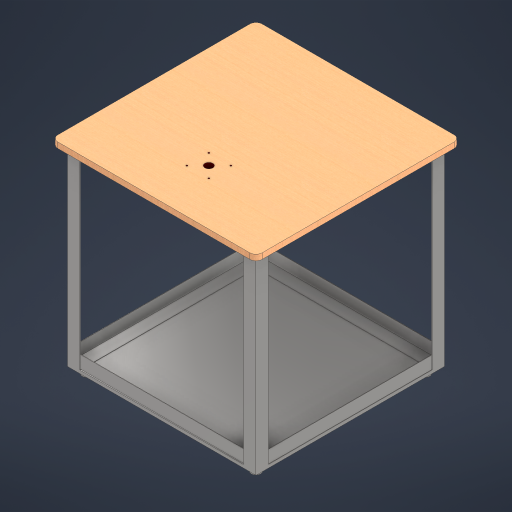
# Autodesk Inventor part: Foundation-Base
Saved by Autodesk Inventor 2023 (Build 270158000, 158)
## iProperties
Created: 2023-09-14
Part Number: Foundation-Base
Material: Steel, Mild
Document SubType Name: Modeling
Designer: Abhinav
Density: 7.85 g/cm^3
Appearance: Semi-Polished
Author: Abhinav
Autodesk Inventor part; units mm, degrees
ref_plane "YZ Plane" through (0, 0, 0) normal (1, 0, 0) x (0, 1, 0)
ref_plane "XZ Plane" through (0, 0, 0) normal (0, 1, 0) x (-1, 0, 0)
ref_plane "XY Plane" through (0, 0, 0) normal (0, 0, 1) x (1, 0, 0)
sketch "Sketch1" plane through (0, 0, 0) normal (0, 1, 0) x (-1, 0, 0)
  line L0 (300, 300) -> (-300, 300)
  line L1 (-300, 300) -> (-300, -300)
  line L2 (-300, -300) -> (300, -300)
  line L3 (300, -300) -> (300, 300)
  line L4 (300, 300) -> (-300, -300) construction
  line L5 (-300, 300) -> (300, -300) construction
  line L6 (-300, 300) -> (-260, 300)
  line L7 (-260, 300) -> (-260, 298.5)
  line L8 (-260, 298.5) -> (-298.5, 298.5)
  line L9 (-300, 298.5) -> (-300, 300)
  line L10 (-300, 300) -> (-298.5, 300)
  line L11 (-298.5, 298.5) -> (-298.5, 260)
  line L12 (-298.5, 260) -> (-300, 260)
  line L13 (-300, 260) -> (-300, 300)
  line L14 (300, 0) -> (0, 0) construction
  line L15 (0, 300) -> (0, 0) construction
  line L16 (300, 300) -> (260, 300)
  line L17 (260, 300) -> (260, 298.5)
  line L18 (260, 298.5) -> (298.5, 298.5)
  line L19 (300, 298.5) -> (300, 300)
  line L20 (300, 300) -> (298.5, 300)
  line L21 (298.5, 298.5) -> (298.5, 260)
  line L22 (298.5, 260) -> (300, 260)
  line L23 (300, 260) -> (300, 300)
  line L24 (300, -300) -> (-300, -300)
  line L25 (-300, -300) -> (-260, -300)
  line L26 (-260, -300) -> (-260, -298.5)
  line L27 (-260, -298.5) -> (-298.5, -298.5)
  line L28 (-300, -298.5) -> (-300, -300)
  line L29 (-300, -300) -> (-298.5, -300)
  line L30 (-298.5, -298.5) -> (-298.5, -260)
  line L31 (-298.5, -260) -> (-300, -260)
  line L32 (-300, -260) -> (-300, -300)
  line L33 (300, -300) -> (298.5, -300)
  line L34 (298.5, -298.5) -> (298.5, -260)
  line L35 (298.5, -260) -> (300, -260)
  line L36 (260, -300) -> (260, -298.5)
  line L37 (260, -298.5) -> (298.5, -298.5)
  line L38 (300, -300) -> (260, -300)
  line L39 (300, -298.5) -> (300, -300)
  line L40 (300, -260) -> (300, -300)
  line L41 (0, 300) -> (0, 150) construction
  circle A0 centre (0, 150) radius 12.5
  line L42 (325, -325) -> (-325, -325)
  line L43 (-325, -325) -> (-325, 325)
  line L44 (-325, 325) -> (325, 325)
  line L45 (325, 325) -> (325, -325)
  line L46 (325, -325) -> (-325, 325) construction
  line L47 (-325, -325) -> (325, 325) construction
  line L48 (35, 185) -> (-35, 185) construction
  line L49 (-35, 185) -> (-35, 115) construction
  line L50 (-35, 115) -> (35, 115) construction
  line L51 (35, 115) -> (35, 185) construction
  line L52 (35, 185) -> (-35, 115) construction
  line L53 (-35, 185) -> (35, 115) construction
  circle A1 centre (35, 115) radius 2.5
  circle A2 centre (-35, 115) radius 2.5
  circle A3 centre (-35, 185) radius 2.5
  circle A4 centre (35, 185) radius 2.5
  point P0 (0, -300)
  dimension "d0" = 600
  dimension "d1" = 600
  dimension "d2" = 40
  dimension "d3" = 1.5
  dimension "d26" = 150
  dimension "d27" = 25
  dimension "d35" = 650
  dimension "d36" = 650
  dimension "d37" = 70
  dimension "d38" = 70
  dimension "d39" = 5
  constraints: 108 end point, 22 symmetric about line, 10 parallel, 9 midpoint, 8 perpendicular, 6 horizontal, 5 centre point, 5 coincident, 3 equal radius
  measures "d0" distance of L2.end L1.end
  measures "d1" distance of L1.end L0.end
  measures "d2" distance of L7.end L9.start
  measures "d3" distance of L6.end L7.end
  measures "d26" distance of L15.start L41.end
  measures "d27" diameter of A0
  measures "d35" distance of L43.end L44.end
  measures "d36" distance of L42.end L43.end
  measures "d37" distance of L50.end L49.end
  measures "d38" distance of L49.end L48.end
  measures "d39" diameter of A1
extrude "Extrusion1" add sketch "Sketch1" along normal blind 18 contours L3 L22 L21 L18 L17 L0 | L17 L18 L21 L22 L3 L35 L34 L37 L36 L2 L26 L27 L30 L31 L1 L12 L11 L8 L7 L0 | L7 L8 L11 L12 L1 L0 | L3 L2 L36 L37 L34 L35 | L31 L30 L27 L26 L2 L1 | L42 L43 L44 L45
extrude "Extrusion2" add sketch "Sketch1" against normal blind 600 contours L3 L22 L21 L18 L17 L0 | L7 L8 L11 L12 L1 L0 | L3 L2 L36 L37 L34 L35 | L31 L30 L27 L26 L2 L1
sketch "Sketch2" plane through (-260, 0, 298.5) normal (0, 0, -1) x (-1, 0, 0)
  line L0 (38.5, -600) -> (-1.5, -600)
  line L1 (-1.5, -600) -> (-1.5, -598.5)
  line L2 (-1.5, -598.5) -> (37, -598.5)
  line L3 (38.5, -598.5) -> (38.5, -600)
  line L4 (38.5, -600) -> (37, -600)
  line L5 (37, -598.5) -> (37, -560)
  line L6 (37, -560) -> (38.5, -560)
  line L7 (38.5, -560) -> (38.5, -600)
  line L8 (-557, -560) -> (-558.5, -560)
  line L9 (-557, -598.5) -> (-557, -560)
  line L10 (-518.5, -598.5) -> (-557, -598.5)
  line L11 (-558.5, -600) -> (-557, -600)
  line L12 (-558.5, -600) -> (-518.5, -600)
  line L13 (-518.5, -600) -> (-518.5, -598.5)
  line L14 (-558.5, -560) -> (-558.5, -600)
  point P0 (-260, 0)
  point P1 (38.5, -600)
  dimension "d11" = 40
  dimension "d12" = 1.5
  constraints: 30 end point, 5 perpendicular, 4 parallel
  measures "d11" distance of L2.start L3.start
  measures "d12" distance of L0.end L2.start
extrude "Extrusion3" add sketch "Sketch2" along normal up to surface (597 mm away)
sketch "Sketch3" plane through (297, -598.5, -298.5) normal (-1, 0, 0) x (0, 0, 1)
  line L0 (0, 0) -> (1.5, 0)
  line L1 (1.5, 1.5) -> (1.5, 40)
  line L2 (1.5, 40) -> (0, 40)
  line L3 (40, 0) -> (40, 1.5)
  line L4 (40, 1.5) -> (1.5, 1.5)
  line L5 (0, 0) -> (40, 0)
  line L6 (0, 1.5) -> (0, 0)
  line L7 (0, 40) -> (0, 0)
  line L8 (557, 1.5) -> (557, 0)
  line L9 (597, 40) -> (595.5, 40)
  line L10 (595.5, 1.5) -> (557, 1.5)
  line L11 (595.5, 40) -> (595.5, 1.5)
  line L12 (597, 0) -> (597, 40)
  line L13 (557, 0) -> (597, 0)
  line L14 (595.5, 0) -> (597, 0)
  line L15 (597, 0) -> (597, 1.5)
  point P0 (298.5, 598.5)
  point P1 (597, 0)
  constraints: 32 end point
extrude "Extrusion4" add sketch "Sketch3" along normal up to surface (594 mm away)
sketch "Sketch4" plane through (0, -600, 0) normal (0, -1, 0) x (1, 0, 0)
  line L0 (-300, -260) -> (-300, -300) projected
  line L1 (300, 300) -> (-300, 300)
  line L2 (-300, 300) -> (-300, -300)
  line L3 (-300, -300) -> (300, -300)
  line L4 (300, -300) -> (300, 300)
  point P0 (0, 0)
  point P1 (-300, -260)
  constraints: 8 end point, 2 parallel, 1 horizontal, 1 perpendicular
extrude "Extrusion5" add sketch "Sketch4" along normal blind 10
sketch "Sketch5" plane through (0, -610, 0) normal (0, -1, 0) x (1, 0, 0)
  circle A0 centre (0, 0) radius 10 projected
  line L0 (0, 0) -> (268.7006, -268.7006) construction
  circle A1 centre (268.7006, -268.7006) radius 15
  line L1 (0, 0) -> (0, -300) construction
  line L2 (260, -300) -> (-260, -300) construction
  circle A2 centre (-268.7006, -268.7006) radius 15
  line L3 (0, 0) -> (-300, 0) construction
  line L4 (-300, -260) -> (-300, 260) construction
  circle A3 centre (268.7006, 268.7006) radius 15
  circle A4 centre (-268.7006, 268.7006) radius 15
  point P0 (0, 0)
  dimension "d21" = 380
  dimension "d22" = 30
  constraints: 6 end point, 4 centre point, 4 symmetric about line, 2 coincident, 2 midpoint, 3 other
  measures "d21" distance of L0.start L0.end
  measures "d22" diameter of A1
extrude "Extrusion6" add sketch "Sketch5" along normal blind 20 contours A1 | A2 | A3 | A4
sketch "Sketch6" plane through (0, 0, 0) normal (0, -1, 0) x (1, 0, 0)
  circle A0 centre (0, 150) radius 12.5 projected
  circle A1 centre (0, 150) radius 105
  point P0 (0, 0)
  dimension "d28" = 210
  constraints: 1 centre point, 1 coincident
  measures "d28" diameter of A1
sketch "Sketch7" plane through (0, 0, 0) normal (0, -1, 0) x (1, 0, 0)
  circle A0 centre (0, 150) radius 12.5 construction
  line L0 (0, 150) -> (0, -250) construction
  line L1 (-30, -273.6478) -> (30, -273.6478) construction
  line L2 (60, -273.6478) -> (60, -213.6478) construction
  line L3 (47.5, -243.6478) -> (47.5, -228.6478) construction
  line L4 (35, -213.6478) -> (60, -213.6478) construction
  line L5 (47.5, -243.6478) -> (47.5, -258.6478) construction
  circle A1 centre (47.5, -228.6478) radius 2.5
  circle A2 centre (47.5, -258.6478) radius 2.5
  line L6 (30, -213.6478) -> (30, -273.6478)
  line L7 (30, -273.6478) -> (60, -273.6478)
  line L8 (60, -213.6478) -> (60, -273.6478)
  line L9 (30, -213.6478) -> (60, -213.6478)
  line L10 (-30, -273.6478) -> (-30, -213.6478)
  line L11 (-30, -213.6478) -> (-60, -213.6478)
  line L12 (-60, -213.6478) -> (-60, -273.6478)
  line L13 (-60, -273.6478) -> (-30, -273.6478)
  line L14 (30, -213.6478) -> (30, -273.6478)
  line L15 (30, -273.6478) -> (30, -213.6478)
  line L16 (35, -213.6478) -> (35, -273.6478)
  line L17 (60, -213.6478) -> (60, -273.6478)
  line L18 (60, -273.6478) -> (35, -273.6478)
  line L19 (35, -273.6478) -> (35, -213.6478)
  line L20 (35, -213.6478) -> (60, -213.6478)
  line L21 (60, -213.6478) -> (35, -273.6478) construction
  line L22 (47.5, -243.6478) -> (60, -243.6478) construction
  circle A3 centre (-47.5, -258.6478) radius 2.5
  line L23 (-35, -273.6478) -> (-60, -273.6478)
  line L24 (-47.5, -243.6478) -> (-47.5, -258.6478) construction
  line L25 (-60, -273.6478) -> (-60, -213.6478)
  line L26 (-35, -213.6478) -> (-60, -273.6478) construction
  line L27 (-35, -213.6478) -> (-35, -273.6478)
  line L28 (-47.5, -243.6478) -> (-47.5, -228.6478) construction
  circle A4 centre (-47.5, -228.6478) radius 2.5
  line L29 (-60, -213.6478) -> (-35, -213.6478)
  line L30 (-47.5, -243.6478) -> (-35, -243.6478) construction
  point P0 (0, 0)
  point P1 (0, -243.6478)
  dimension "d31" = 400
  dimension "d41" = 15
  dimension "d42" = 5
  dimension "d43" = 15
  dimension "d44" = 5
  constraints: 62 end point, 7 equal length, 4 centre point, 4 coincident, 4 midpoint, 4 perpendicular, 2 collinear, 2 equal radius, 1 vertical
  measures "d31" distance of L0.start L0.end
  measures "d41" distance of L3.start L3.end
  measures "d42" diameter of A1
  measures "d43" distance of L24.start L28.end
  measures "d44" diameter of A4
extrude "Extrusion8" cut sketch "Sketch7" against normal blind 10 contours A1 | A2 | A3 | A4
fillet "Fillet1" radius 20 4 edges at (325, 9, 325) (-325, 9, 325) (325, 9, -325) (-325, 9, -325)
body "Solid1"
